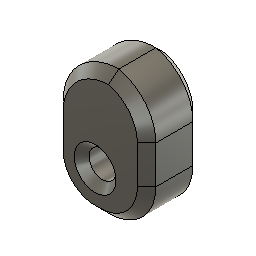
fix_casque_JBL_v2 (Autodesk Fusion 360 design; units mm, degrees)
Autodesk Fusion 360 part; units mm, degrees
note: some values were not read from the file. Set by a fixed rule: which sketch regions a step uses.
sketch "Sketch1" plane through (0, 0, 0) normal (0, 0, 1) x (1, 0, 0)
  circle A0 centre (0, 0) radius 0.725
  circle A1 centre (0, 0) radius 2.225
  line L0 (-2.2249, -0.0244) -> (3.7751, -0.0244)
  line L1 (0, 0) -> (0, -2.225)
  line L2 (0, -2.225) -> (3.7751, -2.225)
  line L3 (3.7751, -2.225) -> (3.7751, -0.0244)
  line L4 (0, -2.225) -> (0, 4.775)
  line L5 (-2.2249, -0.0244) -> (-2.2249, 4.775)
  line L6 (-2.2249, 4.775) -> (0, 4.775)
  line L7 (3.7751, -0.0244) -> (3.7751, 4.775)
  line L8 (3.7751, 4.775) -> (0, 4.775)
  line L9 (3.7751, -2.225) -> (2.7751, -2.225)
  line L10 (2.7751, -2.225) -> (2.7751, 4.775)
  dimension "d1" = 1.45
  dimension "d2" = 4.45
  dimension "d4" = 6
  dimension "d5" = 7
  dimension "d12" = 1
  constraint coincident A0.centre A1.centre
  constraint coincident A1 L0.start
  constraint coincident A1 L1.end
  constraint perpendicular L0 L1
  constraint tangent A1 L2
  constraint perpendicular L0 L3
  constraint perpendicular L0 L4
  constraint perpendicular L0 L5
  constraint perpendicular L4 L6
  constraint perpendicular L6 L7
  constraint perpendicular L4 L8
  constraint perpendicular L3 L9
  constraint coincident L8 L10.end
  constraint perpendicular L8 L10
  measures "d1" diameter of A0
  measures "d2" diameter of A1
  measures "d4" distance of L0.start L0.end
  measures "d5" distance of L1.end L4.end
  measures "d12" distance of L2.end L9.end
extrude "Extrude1" add sketch "Sketch1" along normal blind 3 contours A0 A1 L0 L4 | A0 A1 L0 L4 | A0 A1 L0 L1 L4 | A0 A1 L0 L1 L4 | A1 L0 L4 L8 L10 | A1 L4 L5 L6 | A1 L0 L2 L10
chamfer "Chamfer2" distance 0.4 angle 45 2 edges at (-0.6759, 0.2622, 3) (-0.6759, 0.2622, 0)
fillet "Fillet2" radius 3 1 edges at (-2.2249, 4.775, 1.5)
fillet "Fillet3" radius 2.5 2 edges at (2.7751, 4.775, 1.5) (2.7751, -2.225, 1.5)
chamfer "Chamfer3" distance 0.5 angle 45 14 edges at (2.2116, 3.9066, 0) (-1.5647, -1.5819, 0) (0.1376, -2.225, 0) (2.0429, -1.4928, 0) (2.7751, 1.3003, 0) (-1.3462, 3.8963, 0) (-2.2249, 0.8753, 0) (-1.3462, 3.8963, 3) (-2.2249, 0.8753, 3) (2.2116, 3.9066, 3) (2.7751, 1.3003, 3) (2.0429, -1.4928, 3) (0.1376, -2.225, 3) (-1.5647, -1.5819, 3)
